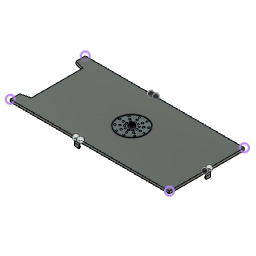
coolingpadcap - Copy v17 (Autodesk Fusion 360 design; units mm, degrees)
Autodesk Fusion 360 part; units mm, degrees
sketch "Sketch1" plane through (0, 0, 0) normal (1, 0, 0) x (0, 1, 0)
sketch "Sketch2" plane through (0, 0, 0) normal (0, 1, 0) x (1, 0, 0)
sketch "Sketch3" plane through (0, 0, 0) normal (0, 0, 1) x (1, 0, 0)
  line L0 (-89.6492, -40) -> (80, -40)
  line L1 (80, -40) -> (80, 40)
  line L2 (80, 40) -> (-89.6492, 40)
  line L3 (-89.6492, 40) -> (-89.6492, 30)
  line L4 (-89.6492, -40) -> (-89.6492, -30)
  line L5 (-89.6492, -40) -> (-79.6492, -40)
  line L6 (-79.6492, 27.5) -> (-79.6492, -27.5)
  line L7 (-79.6492, 27.5) -> (-89.6492, 30)
  line L8 (-89.6492, -30) -> (-79.6492, -27.5)
  constraint horizontal L0
  constraint perpendicular L0 L1
  constraint perpendicular L1 L2
  constraint coincident L0 L5.end
extrude "Extrude1" add sketch "Sketch3" along normal blind 2.5 makes body 1
sketch "Sketch4" plane through (0, 0, 2.5) normal (0, 0, 1) x (-1, 0, 0)
  line L0 (-80, 40) -> (-80, -40)
  line L1 (89.6492, -40) -> (89.6492, -30)
  line L2 (89.6492, -30) -> (79.6492, -27.5)
  line L3 (79.6492, -27.5) -> (79.6492, 27.5)
  line L4 (79.6492, 27.5) -> (89.6492, 30)
  line L5 (89.6492, 30) -> (89.6492, 40)
sketch "Sketch5" plane through (0, 0, 2.5) normal (0, 0, 1) x (-1, 0, 0)
  line L0 (89.6492, 40) -> (-80, 40)
  line L1 (-80, 40) -> (-80, -40)
  line L2 (-80, -40) -> (89.6492, -40)
  line L3 (89.6492, -40) -> (89.6492, -30)
  line L4 (89.6492, -30) -> (79.6492, -27.5)
  line L5 (79.6492, -27.5) -> (79.6492, 27.5)
  line L6 (79.6492, 27.5) -> (89.6492, 30)
  line L7 (89.6492, 30) -> (89.6492, 40)
  line L8 (19.6492, 40) -> (14.6492, 40)
  line L9 (19.6492, -40) -> (14.6492, -40)
  line L10 (-80, 2.5) -> (-80, -2.5)
  dimension "d16" = 5
  dimension "d18" = 5
  dimension "d20" = 5
  constraint perpendicular L7 L8
  constraint coincident L2 L9.start
  constraint coincident L2 L9.end
  constraint coincident L1 L10.start
  constraint perpendicular L0 L10
  measures "d16" distance of L8.start L8.end
  measures "d18" distance of L9.start L9.end
  measures "d20" distance of L10.start L10.end
sketch "Sketch6" plane through (0, 0, 0) normal (1, 0, 0) x (0, 1, 0)
  line L0 (-40.5, 2.5) -> (-40.8, 2.5)
  line L1 (-40.8, 2.5) -> (-40.8, 2.4)
  line L2 (-40.8, 2.4) -> (-40.5, 2.4)
  line L3 (-40.5, 2.4) -> (-40.5, 2.5)
  constraint horizontal L0
  constraint vertical L1
  constraint horizontal L2
  constraint vertical L3
extrude "Extrude2" add sketch "Sketch6" along normal blind 5 separate body makes body 2
move_body "Move1" bodies 2 to x (1, 0, 0) y (0, 1, 0) z (0, 0, 1) at (-20, 0, 0)
move_body "Move2" bodies 2 to x (1, 0, 0) y (0, 1, 0) z (0, 0, 1) at (0.35, 0, 0)
extrude "Extrude3" add 1 faces at (-16.3167, -40.7, 2.4) along direction (0, 0, -1) blind 2.4 on bodies 2 bodies 2
sketch "Sketch7" plane through (-19.65, 0, 0) normal (-1, 0, 0) x (0, -1, 0)
  line L0 (40.5, 2.5) -> (40.5, 0)
  line L1 (40.5, 0) -> (40.8, 0)
  line L2 (40.8, 0) -> (40.8, 2.5)
  line L3 (40.8, 2.5) -> (40.5, 2.5)
  line L4 (40.8, 0) -> (40.8, -3)
  line L5 (40.8, -3) -> (40.8, -5)
  line L6 (40.8, -5) -> (39.3381, -3.2333)
  line L7 (39.3381, -3.2333) -> (40.303, -2.4349)
  line L8 (40.303, -2.4349) -> (40.303, 0)
  line L9 (40.303, 0) -> (40.8, 0)
  constraint coincident L1.end L2.start
  constraint perpendicular L1 L4
  constraint perpendicular L1 L5
  constraint perpendicular L6 L7
  constraint parallel L5 L8
extrude "Extrude4" add sketch "Sketch7" against normal blind 5 contours L1 L4 L5 L6 L7 L8 L9 bodies 2
move_body "Move3" bodies 2 to x (1, 0, 0) y (0, 1, 0) z (0, 0, 1) at (0, -0.6, 0)
extrude "Extrude5" add 1 faces at (-16.3167, -41.1, 1.6667) along direction (0, 1, 0) blind 1.1 separate body on bodies 2 makes body 3
move_body "Move4" bodies 2 3 to x (1, 0, 0) y (0, 1, 0) z (0, 0, 1) at (0, -1.5, 0)
copy_body "Body->Comp1" bodies 2 removing the originals makes body 4 in component "Component"
copy_body "Body->Comp2" bodies 3 removing the originals makes body 5 in component "Component'"
copy_body "CopyPasteBodies1" bodies 5 4 makes body 6 makes body 7
move_body "Move5" bodies 6 7 to x (-1, 0, 0) y (0, -1, 0) z (0, 0, 1) at (-34.3, -1.2, 0)
copy_body "CopyPasteBodies2" bodies 4 5 makes body 8 makes body 9
move_body "Move6" bodies 8 9 to x (0, 1, 0) y (-1, 0, 0) z (0, 0, 1) at (38.947, 17.147, 0)
move_body "Move1'" bodies 4 to x (1, 0, 0) y (0, 1, 0) z (0, 0, 1) at (0, 1.5, 0) in component "Component"
move_body "Move1''" bodies 5 to x (1, 0, 0) y (0, 1, 0) z (0, 0, 1) at (0, 1.5, 0) in component "Component'"
move_body "Move7" bodies 8 9 to x (1, 0, 0) y (0, 1, 0) z (0, 0, 1) at (-0.4, 0, 0)
move_body "Move8" bodies 6 7 to x (1, 0, 0) y (0, 1, 0) z (0, 0, 1) at (0, -0.3, 0)
sketch "Sketch8" plane through (0, 0, 0) normal (0, 0, -1) x (1, 0, 0)
  line L0 (80, 40) -> (-89.6492, 40)
  line L1 (-89.6492, 40) -> (-89.6492, 30)
  line L2 (-89.6492, 30) -> (-79.6492, 27.5)
  line L3 (-79.6492, 27.5) -> (-79.6492, -27.5)
  line L4 (-79.6492, -27.5) -> (-89.6492, -30)
  line L5 (-89.6492, -30) -> (-89.6492, -40)
  line L6 (-89.6492, -40) -> (80, -40)
  line L7 (80, -40) -> (80, 40)
  circle A0 centre (0, 0) radius 15
  circle A1 centre (2, 0) radius 1
  circle A2 centre (5.5552, 0) radius 1
  circle A3 centre (9, 0) radius 1
  circle A4 centre (13, 0) radius 1
  dimension "d29" = 30
  dimension "d30" = 2
  dimension "d31" = 2
  dimension "d32" = 2
  dimension "d33" = 2
  constraint coincident A0.centre origin
  measures "d29" diameter of A0
  measures "d30" diameter of A1
  measures "d31" diameter of A2
  measures "d32" diameter of A3
  measures "d33" diameter of A4
extrude "Extrude6" cut sketch "Sketch8" against normal blind 4 contours A1 | A2 | A3 | A4 bodies 1
sketch "Sketch9" plane through (0, 0, 2.5) normal (0, 0, 1) x (-1, 0, 0)
  circle A0 centre (0, 0) radius 15
  dimension "d36" = 30
  constraint coincident A0.centre origin
  measures "d36" diameter of A0
pattern_circular "C-Pattern1" count 10 over 360 about axis through (0, 0, 2.5) along (0, 0, 1) of 3 faces at (13.995, 0.0996, 0.8333) (9.995, 0.0996, 0.8333) (6.5503, 0.0996, 0.8333) on bodies 1
pattern_circular "C-Pattern2" count 5 over 360 about axis through (0, 0, 2.5) along (0, 0, 1) of 1 faces at (2.995, 0.0996, 0.8333) on bodies 1
copy_body "Body->Comp3" bodies 7 removing the originals makes body 10 in component "Component''"
copy_body "Body->Comp4" bodies 1 removing the originals makes body 11 in component "Component'''"
copy_body "Body->Comp5" bodies 9 removing the originals makes body 12 in component "Component''''"
copy_body "Body->Comp1'" bodies 4 removing the originals makes body 13 in component "Component'''''"
copy_body "Body->Comp1''" bodies 5 removing the originals makes body 14 in component "Component''''''"
copy_body "Body->Comp6" bodies 6 removing the originals makes body 15 in component "Component'''''''"
copy_body "Body->Comp7" bodies 8 removing the originals makes body 16 in component "Component''''''''"
component "Component" placed x (1, 0, 0) y (0, 1, 0) z (0, 0, 1) at (0, 0, 0)
component "Component'" placed x (1, 0, 0) y (0, 1, 0) z (0, 0, 1) at (0, 0, 0)
component "Component''" placed x (1, 0, 0) y (0, 1, 0) z (0, 0, 1) at (0, 0, 0)
component "Component'''" placed x (1, 0, 0) y (0, 1, 0) z (0, 0, 1) at (0, 0, 0)
component "Component''''" placed x (1, 0, 0) y (0, 1, 0) z (0, 0, 1) at (0, 0, 0)
component "Component'''''''" placed x (1, 0, 0) y (0, 1, 0) z (0, 0, 1) at (0, 0, 0)
component "Component''''''''" placed x (1, 0, 0) y (0, 1, 0) z (0, 0, 1) at (0, 0, 0)
component "Component'''''" placed x (1, 0, 0) y (0, 1, 0) z (0, 0, 1) at (0, 0, 0) in component "Component"
component "Component''''''" placed x (1, 0, 0) y (0, 1, 0) z (0, 0, 1) at (0, 0, 0) in component "Component'"
